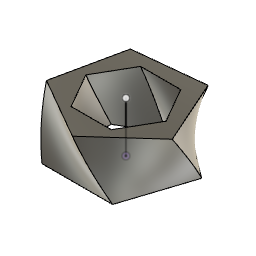
proj2-main (Autodesk Fusion 360 design; units mm, degrees)
Autodesk Fusion 360 part; units mm, degrees
sketch "草图1" plane through (0, 0, 0) normal (0, 0, 1) x (1, 0, 0)
  line L0 (14.2658, 4.6353) -> (0, 15)
  line L1 (0, 15) -> (-14.2658, 4.6353)
  line L2 (-14.2658, 4.6353) -> (-8.8168, -12.1353)
  line L3 (-8.8168, -12.1353) -> (8.8168, -12.1353)
  line L4 (8.8168, -12.1353) -> (14.2658, 4.6353)
sketch "草图2" plane through (0, 0, 0) normal (0, 0, 1) x (1, 0, 0)
  line L0 (0, 10) -> (-8.6603, 5)
  line L1 (-8.6603, 5) -> (-8.6603, -5)
  line L2 (-8.6603, -5) -> (0, -10)
  line L3 (0, -10) -> (8.6603, -5)
  line L4 (8.6603, -5) -> (8.6603, 5)
  line L5 (8.6603, 5) -> (0, 10)
form "造型1" [no effect]
sketch "草图3" plane through (0, 0, 0) normal (1, 0, 0) x (0, 1, 0)
  line L0 (0, 0) -> (0, 12.5)
  constraint coincident L0.start origin
  constraint vertical L0
sweep "扫掠1" add twist angle -30 profiles "草图1" path "草图3" along L0 section 1
sweep "扫掠2" cut twist angle 30 profiles "草图2" path "草图3" along L0 section 1
